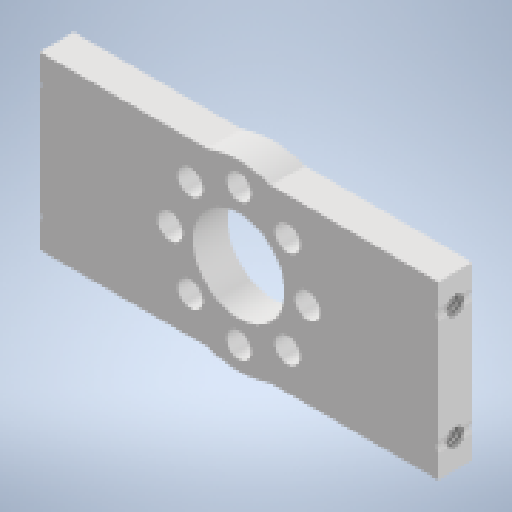
# Autodesk Inventor part: udeyi
Saved by Autodesk Inventor 2024 (Build 280153000, 153)
## iProperties
Created: 2023-12-31
Part Number: udeyi
Material: 一般
Document SubType Name: Modeling
Designer: right
Density: 1 g/cm^3
Appearance: 既定
Author: right
Autodesk Inventor part; units mm, degrees
ref_plane "YZ Plane" through (0, 0, 0) normal (1, 0, 0) x (0, 1, 0)
ref_plane "XZ Plane" through (0, 0, 0) normal (0, 1, 0) x (-1, 0, 0)
ref_plane "XY Plane" through (0, 0, 0) normal (0, 0, 1) x (1, 0, 0)
sketch "スケッチ1" plane through (0, 0, 0) normal (0, 0, 1) x (1, 0, 0)
  circle A0 centre (0, 0) radius 4
  circle A1 centre (0, 0) radius 8
  circle A2 centre (0, 0) radius 6 construction
  circle A3 centre (0, 6) radius 1.1
  circle A4 centre (-4.2426, 4.2426) radius 1.1
  circle A5 centre (-6, 0) radius 1.1
  circle A6 centre (-4.2426, -4.2426) radius 1.1
  circle A7 centre (0, -6) radius 1.1
  circle A8 centre (4.2426, -4.2426) radius 1.1
  circle A9 centre (6, 0) radius 1.1
  circle A10 centre (4.2426, 4.2426) radius 1.1
  line L0 (-17.45, -7.5) -> (17.45, -7.5)
  line L1 (17.45, -7.5) -> (17.45, 7.5)
  line L2 (17.45, 7.5) -> (-17.45, 7.5)
  line L3 (-17.45, 7.5) -> (-17.45, -7.5)
  line L4 (-17.45, -7.5) -> (17.45, 7.5) construction
  line L5 (17.45, -7.5) -> (-17.45, 7.5) construction
  point P0 (2.7839, 7.5)
  point P1 (-2.7839, 7.5)
  point P2 (2.7839, -7.5)
  point P3 (-2.7839, -7.5)
  dimension "d2" = 12
  dimension "d0" = 8
  dimension "d1" = 16
  dimension "d3" = 2.2
  dimension "d6" = 360
  dimension "d8" = 34.9
  dimension "d9" = 15
  constraints: 12 end point, 10 centre point, 3 coincident, 2 midpoint, 2 parallel, 2 vertical alignment, 1 horizontal, 1 perpendicular, 19 other
  measures "d0" diameter of A0
  measures "d1" diameter of A1
  measures "d3" diameter of A3
  measures "d8" distance of L1.end L2.end
  measures "d9" distance of L0.end L1.end
extrude "押し出し1" add sketch "スケッチ1" along normal blind 3
sketch "スケッチ2" plane through (17.45, -7.5, 0) normal (1, 0, 0) x (0, 0, -1)
  line L0 (0, 7.5) -> (-3, 7.5) construction
  line L1 (-3, 0) -> (-3, 15) construction
  line L2 (-1.5, 7.5) -> (-1.5, 15) construction
  line L3 (0, 15) -> (-3, 15) construction
  point P0 (-1.5, 12.5)
  point P1 (-1.5, 2.5)
  dimension "d12" = 5
  constraints: 4 end point, 3 midpoint, 1 point on line, 1 symmetric about line
  measures "d12" distance from line of L0 point (-1.5, 12.5)
hole "穴1" at (17.45, 5, 1.5) at (17.45, -5, 1.5) direction (-1, 0, 0) diameter 1.567 depth 4.5 tip angle 118 thread size "M2x0.4" class "6H" standard "ISO Metric profile"
sketch "スケッチ3" plane through (-17.45, -7.5, 0) normal (-1, 0, 0) x (0, 0, 1)
  circle A0 centre (1.5, 2.5) radius 0.7835 projected
  circle A1 centre (1.5, 12.5) radius 0.7835 projected
  point P0 (0, 7.5)
  point P1 (1.5, 2.5)
  point P2 (1.5, 12.5)
  constraints: 2 coincident
hole "穴2" at (-17.45, -5, 1.5) at (-17.45, 5, 1.5) direction (1, 0, 0) diameter 1.567 depth 4.5 tip angle 118 thread size "M2x0.4" class "6H" standard "ISO Metric profile"
sketch "スケッチ4" plane through (0, 0, 0) normal (0, 0, -1) x (-1, 0, 0)
  line L0 (17.45, -4.2165) -> (17.45, -5.7835) projected
  circle A0 centre (0, -6) radius 1.1 projected
  line L1 (0, -6) -> (0, 0) construction
  circle A1 centre (18.45, -5) radius 1.1
  circle A2 centre (6, 0) radius 1.1 construction
  line L2 (0, 0) -> (6, 0) construction
  circle A3 centre (18.45, 5) radius 1.1
  line L3 (-17.45, -4.2165) -> (-17.45, -5.7835)
  circle A4 centre (-18.45, -5) radius 1.1
  circle A5 centre (-18.45, 5) radius 1.1
  point P0 (17.45, -5)
  point P1 (-17.45, -5)
  dimension "d27" = 2.2
  dimension "d28" = 1
  constraints: 6 end point, 6 symmetric about line, 4 centre point, 1 horizontal, 1 horizontal alignment, 1 midpoint, 1 vertical, 3 other
  measures "d27" diameter of A1
  measures "d28" distance from line of L0 A1.centre
extrude "押し出し2" cut sketch "スケッチ4" against normal blind 3 contours A1 L0 | L0 A1 | A3 | A4 L3 | L3 A4 | A5
